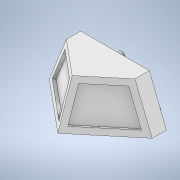
# Autodesk Inventor part: Vasilecowcatcher
Saved by Autodesk Inventor 2020 (Build 240168000, 168)
## iProperties
Created: 2020-04-30
Part Number: Vasilecowcatcher
Material: ABS Plastic
Document SubType Name: Modeling
Designer: al
Density: 1.06 g/cm^3
Appearance: Smooth - White
Author: al
Autodesk Inventor part; units mm, degrees
ref_plane "YZ Plane" through (0, 0, 0) normal (1, 0, 0) x (0, 1, 0)
ref_plane "XZ Plane" through (0, 0, 0) normal (0, 1, 0) x (-1, 0, 0)
sketch "Sketch1" plane through (0, 0, 0) normal (0, 0, 1) x (1, 0, 0)
  line L0 (0, 0) -> (45.72, 0)
  line L1 (45.72, 0) -> (45.72, 6.35)
  line L2 (0, 0) -> (0, 6.35)
  line L3 (45.72, 6.35) -> (22.86, 25.4)
  line L4 (22.86, 25.4) -> (0, 6.35)
  dimension "d0" = 45.72
  dimension "d1" = 6.35
  dimension "d2" = 6.35
  dimension "d3" = 25.4
  dimension "d4" = 22.86
  constraints: 10 end point, 2 vertical, 1 horizontal
  measures "d0" distance of L0.start L0.end
  measures "d1" distance of L0.end L1.end
  measures "d2" distance of L0.start L2.end
  measures "d3" distance from line of L3.end L0
  measures "d4" distance from line of L3.end L1
ref_plane "Work Plane1" through (0, 0, 19.05) normal (0, 0, 1) x (1, 0, 0)
sketch "Sketch2" plane through (0, 0, 19.05) normal (0, 0, 1) x (1, 0, 0)
  line L0 (22.86, 25.4) -> (0, 6.35) projected
  line L1 (45.72, 6.35) -> (22.86, 25.4) projected
  line L2 (45.72, 0) -> (45.72, 6.35) projected
  line L3 (0, 0) -> (45.72, 0) projected
  line L4 (0, 0) -> (0, 6.35) projected
  line L5 (38.1, 0) -> (7.62, 0)
  line L6 (7.62, 6.35) -> (22.86, 19.05)
  line L7 (22.86, 19.05) -> (38.1, 6.35)
  line L8 (38.1, 6.35) -> (38.1, 0)
  line L9 (7.62, 6.35) -> (7.62, 0)
  dimension "d6" = 6.35
  dimension "d7" = 6.35
  dimension "d9" = 7.62
  dimension "d10" = 7.62
  dimension "d11" = 19.05
  dimension "d12" = 15.24
  constraints: 10 end point, 2 parallel, 2 point on line, 1 perpendicular
  measures "d6" distance of L6.start L5.end
  measures "d7" distance of L7.end L5.start
  measures "d9" distance between parallel lines of L9 L4
  measures "d10" distance between parallel lines of L2 L8
  measures "d11" vertical distance of L6.end L5.start
  measures "d12" distance from line of L6.end L9
loft "Loft1" add profiles "Sketch1", "Sketch2" contours all / L9 L6 L7 L8 L3
shell "Shell1" thickness 2.54 removed faces 1 at (22.86, 8.4667, 0)
sketch "Sketch6" plane through (0, 6.35, 0) normal (-0.6201737, 0.7442084, 0.2480695) x (0.7682213, 0.6401844, 0)
  line L0 (29.7571, 0) -> (25.6919, -19.6647) projected
  line L1 (29.7571, 0) -> (25.6919, -19.6647)
  line L2 (0, 0) -> (5.8538, -19.6647) projected
  line L3 (25.6919, -19.6647) -> (5.8538, -19.6647)
  line L4 (5.8538, -19.6647) -> (0, 0)
  line L5 (0, 0) -> (29.7571, 0)
  line L6 (7.7479, -17.1247) -> (23.6233, -17.1247)
  line L7 (23.6233, -17.1247) -> (26.6383, -2.54)
  line L8 (26.6383, -2.54) -> (3.4063, -2.54)
  line L9 (3.4063, -2.54) -> (7.7479, -17.1247)
  point P0 (-4.0652, -1.2101)
  dimension "d18" = 2.54
  constraints: 16 end point, 2 collinear, 2 parallel, 1 horizontal, 3 other
  measures "d18" distance between parallel lines of L3 L6
extrude "Extrusion1" cut sketch "Sketch6" against normal blind 1.27 contours L9 L8 L7 L6
sketch "Sketch7" plane through (22.86, 25.4, 0) normal (0.6201737, 0.7442084, 0.2480695) x (0.7682213, -0.6401844, 0)
  line L0 (29.7571, 0) -> (23.9032, -19.6647) projected
  line L1 (29.7571, 0) -> (23.9032, -19.6647)
  line L2 (0, 0) -> (4.0652, -19.6647) projected
  line L3 (23.9032, -19.6647) -> (4.0652, -19.6647)
  line L4 (4.0652, -19.6647) -> (0, 0)
  line L5 (0, 0) -> (29.7571, 0)
  line L6 (6.1338, -17.1247) -> (22.0092, -17.1247)
  line L7 (22.0092, -17.1247) -> (26.3508, -2.54)
  line L8 (26.3508, -2.54) -> (3.1188, -2.54)
  line L9 (3.1188, -2.54) -> (6.1338, -17.1247)
  point P0 (-1.3009, -8.4709)
  dimension "d21" = 2.54
  constraints: 16 end point, 2 collinear, 2 parallel, 1 horizontal, 3 other
  measures "d21" distance between parallel lines of L3 L6
extrude "Extrusion2" cut sketch "Sketch7" against normal blind 1.27 contours L9 L8 L7 L6
sketch "Sketch8" plane through (0, 0, 0) normal (0, -1, 0) x (1, 0, 0)
  circle A0 centre (6.985, 3.175) radius 1.5875
  circle A1 centre (22.86, 15.875) radius 1.5835
  circle A2 centre (38.735, 3.175) radius 1.5875
  line L0 (0, 0) -> (45.72, 0) projected
  dimension "d24" = 3.167
  dimension "d25" = 3.175
  dimension "d26" = 3.175
  dimension "d27" = 31.75
  dimension "d28" = 6.985
  dimension "d29" = 15.875
  dimension "d30" = 22.86
  dimension "d31" = 3.175
  dimension "d32" = 3.175
  constraints: 3 centre point
  measures "d24" diameter of A1
  measures "d25" diameter of A2
  measures "d26" diameter of A0
  measures "d27" distance of A2.centre A0.centre
  measures "d28" horizontal distance of L0.start A0.centre
  measures "d29" distance from line of L0 A1.centre
  measures "d30" horizontal distance of L0.end A1.centre
  measures "d31" distance from line of L0 A2.centre
  measures "d32" vertical distance of L0.start A0.centre
extrude "Extrusion3" add sketch "Sketch8" along normal blind 3.175
chamfer "Chamfer1" distance 0.254 angle 45 3 edges at (21.2765, -3.175, 15.875) (37.1475, -3.175, 3.175) (5.3975, -3.175, 3.175)
body "Solid1"
